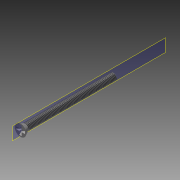
# Autodesk Inventor part: Fi3es60mmcsavar
Saved by Autodesk Inventor 2015 (Build 190159000, 159)
## iProperties
Created: 2014-11-03
Part Number: Fi3es60mmcsavar
Material: Steel, Alloy
Document SubType Name: Modeling
Designer: laca
Density: 7.73 g/cm^3
Appearance: Semi-Polished
Mass: 2.229 g
Surface Area: 4.25731 cm^2
Volume: 0.288357 cm^3
Author: laca
Autodesk Inventor part; units mm, degrees
ref_plane "YZ Plane" through (0, 0, 0) normal (1, 0, 0) x (0, 1, 0)
ref_plane "XZ Plane" through (0, 0, 0) normal (0, 1, 0) x (-1, 0, 0)
ref_plane "XY Plane" through (0, 0, 0) normal (0, 0, 1) x (1, 0, 0)
sketch "Sketch1" plane through (0, 0, 0) normal (0, 1, 0) x (-1, 0, 0)
  line L0 (0, 3.9544) -> (2.5, 3.9544)
  line L1 (2.5, 3.9544) -> (1.5, 1.9544)
  line L2 (1.5, 1.9544) -> (1.5, -36.0456)
  line L3 (1.5, -36.0456) -> (0, -36.0456)
  line L4 (0, -36.0456) -> (0, 3.9544)
  point P0 (0, 0)
  dimension "d0" = 2.5
  dimension "d1" = 2
  dimension "d2" = 40
  dimension "d21" = 1.5
  constraints: 10 end point, 3 perpendicular, 1 horizontal
  measures "d0" distance of L0.start L0.end
  measures "d1" distance from line of L1.end L0
  measures "d2" distance between parallel lines of L3 L0
  measures "d21" distance between parallel lines of L4 L2
revolve "Revolution1" add sketch "Sketch1" angle 360 about axis through (0, 0, -36.0456) along (0, 0, 1)
sketch "Sketch2" plane through (0, 0, 3.9544) normal (0, 0, 1) x (1, 0, 0)
  line L0 (-0.5, 0) -> (0.5, 0)
  line L1 (0.5, 0) -> (0.5, 2)
  line L2 (0.5, 2) -> (-0.5, 2)
  line L3 (-0.5, 2) -> (-0.5, 0)
  point P0 (0, 0)
  dimension "d4" = 1
  dimension "d5" = 2
  dimension "d6" = 0.5
  constraints: 8 end point, 2 parallel, 1 horizontal, 1 horizontal alignment, 1 perpendicular
  measures "d4" distance of L1.end L2.end
  measures "d5" distance of L2.end L0.start
  measures "d6" distance from line of point (0, 0) L3
ref_plane "Work Plane2" through (-0.5, 2, 3.9544) normal (-1, 0, 0) x (0, -1, 0)
sketch "Sketch4" plane through (-0.5, 2, 3.9544) normal (-1, 0, 0) x (0, -1, 0)
  line L0 (-0.5, 0) -> (4.5, 0) projected
  line L1 (-0.4472, 0) -> (0.7164, -1.2393)
  point P0 (2, -3.9544)
  dimension "d15" = 1.7
  constraints: 2 end point, 1 point on line
  measures "d15" distance of L1.start L1.end
sweep "Sweep1" cut profiles "Sketch2" path "Sketch4" path curves L1
pattern_circular "Circular Pattern1" count 4 over 360 about axis through (0, 0, 2.9544) along (0, 0, -1) of "Sweep1"
thread "Thread2"
equation "\"d6\" = 0.5 * d4"
body "Solid1"
